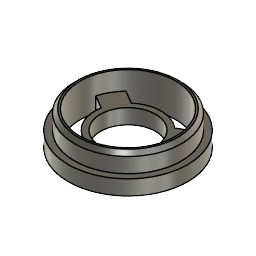
Drill_head_axle_holder (Autodesk Fusion 360 design; units mm, degrees)
Autodesk Fusion 360 part; units mm, degrees
sketch "Skizze1" plane through (0, 0, 0) normal (0, 0, 1) x (1, 0, 0)
  circle A0 centre (0, 0) radius 16
  circle A1 centre (0, 0) radius 14.325
  circle A2 centre (0, 0) radius 12.825
  circle A3 centre (0, 0) radius 7.4
  circle A4 centre (0, 0) radius 8.9
  line L0 (0, -8.9) -> (-2.9249, -8.9)
  line L1 (-2.9249, -8.9) -> (3, -8.9)
  line L2 (-2.9249, -8.9) -> (3, -8.9)
  line L3 (3, -8.9) -> (3, -17.9851)
  line L4 (3, -17.9851) -> (-2.9249, -17.9851)
  line L5 (-2.9249, -17.9851) -> (-2.9249, -8.9)
  line L6 (-2.9249, -8.9) -> (-2.9249, -8.4056)
  line L7 (3, -8.9) -> (3, -8.3791)
  line L8 (6.2076, 7.0481) -> (14.0756, 11.5906)
  line L9 (17.038, 6.4595) -> (9.1701, 1.917)
  line L10 (9.1701, 1.917) -> (8.742, 1.6698)
  line L11 (6.2076, 7.0481) -> (5.7565, 6.7876)
  line L12 (-9.2076, 1.8519) -> (-17.0756, 6.3945)
  line L13 (-14.1131, 11.5256) -> (-6.2452, 6.983)
  line L14 (-6.2452, 6.983) -> (-5.817, 6.7359)
  line L15 (-9.2076, 1.8519) -> (-8.7565, 1.5915)
  dimension "d1" = 32
  dimension "d2" = 28.65
  dimension "d3" = 1.5
  dimension "d4" = 14.8
  dimension "d5" = 1.5
  dimension "d7" = 360
  constraint coincident A0.centre A1.centre
  constraint concentric A0 A1
  constraint concentric A0 A2
  constraint concentric A1 A3
  constraint concentric A2 A4
  constraint coincident A4 L0.start
  constraint tangent A4 L0
  constraint horizontal L0
  constraint parallel L0 L1
  constraint perpendicular L2 L3
  constraint parallel L2 L4
  constraint parallel L3 L5
  constraint coincident A4 L6.end
  constraint perpendicular L2 L6
  constraint coincident A4 L7.end
  constraint perpendicular L2 L7
  measures "d1" diameter of A0
  measures "d2" diameter of A1
  measures "d3" distance of A1 A2
  measures "d4" diameter of A3
  measures "d5" distance of A3 A4
extrude "Extrusion1" add sketch "Skizze1" against normal blind 4 contours A0 A1 L3 L9 | A0 A1 L8 L9 | A0 A1 L3 L5 | A0 A1 L8 L13 | A1 A2 L8 L9 | A1 A2 L3 L9 | A0 A1 L5 L12 | A1 A2 L3 L5 | A0 A1 L12 L13 | A1 A2 L8 L13 | A2 A4 L8 L9 L10 L11 | A1 A2 L5 L12 | A2 L0 L1 L2 L3 L5 | A1 A2 L12 L13 | A4 L1 L2 L7 | A2 A4 L12 L13 L14 L15 | A4 | A4 L0 L1 L2 L6
extrude "Extrusion2" add sketch "Skizze1" along normal blind 5 contours A1 A2 L8 L9 | A1 A2 L3 L9 | A1 A2 L3 L5 | A1 A2 L8 L13 | A1 A2 L5 L12 | A1 A2 L12 L13
chamfer "Fase1" distance 1 angle 45 1 edges at (-13.3556, -5.1801, 5)
extrude "Extrusion3" [suppressed]
move_face "Flächen versetzen1" [suppressed]
equation "d15 = ( ( 14.4 - 8.2 ) / 2 ) * 1 mm"
